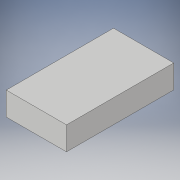
# Autodesk Inventor part: Part1
Saved by Autodesk Inventor 2019.1 (Build 231200000, 200)
## iProperties
Created: 2019-07-15
Part Number: Part1
Material: Generic
Document SubType Name: Modeling
Designer: everton
Density: 1 g/cm^3
Appearance: Default
Author: everton
Autodesk Inventor part; units mm, degrees
ref_plane "YZ Plane" through (0, 0, 0) normal (1, 0, 0) x (0, 1, 0)
ref_plane "XZ Plane" through (0, 0, 0) normal (0, 1, 0) x (-1, 0, 0)
ref_plane "XY Plane" through (0, 0, 0) normal (0, 0, 1) x (1, 0, 0)
sketch "Sketch1" plane through (0, 0, 0) normal (0, 1, 0) x (-1, 0, 0)
  line L0 (6.1363, 8.0276) -> (-9.3306, 8.0276)
  line L1 (-9.3306, 8.0276) -> (-9.3306, -19.5017)
  line L2 (-9.3306, -19.5017) -> (6.1363, -19.5017)
  line L3 (6.1363, -19.5017) -> (6.1363, 8.0276)
  point P0 (0, 0)
  constraints: 8 end point, 2 parallel, 1 horizontal, 1 perpendicular
extrude "Extrusion1" add sketch "Sketch1" along normal blind 6
body "Solid1"
